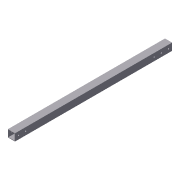
# Autodesk Inventor part: Frame_RearVerticalSupport
Saved by Autodesk Inventor 2012 (Build 160160000, 160)
## iProperties
Created: 2012-01-09
Part Number: Frame_RearVerticalSupport
Material: Aluminum-6061
Document SubType Name: Modeling
Designer: JesseK
Density: 2.71 g/cm^3
Mass: 228.217 g
Surface Area: 1066.35 cm^2
Volume: 84.213 cm^3
Author: JesseK
Autodesk Inventor part; units mm, degrees
ref_plane "YZ Plane" through (0, 0, 0) normal (1, 0, 0) x (0, 1, 0)
ref_plane "XZ Plane" through (0, 0, 0) normal (0, 1, 0) x (-1, 0, 0)
ref_plane "XY Plane" through (0, 0, 0) normal (0, 0, 1) x (1, 0, 0)
sketch "Sketch1" plane through (0, 0, 0) normal (0, 0, 1) x (1, 0, 0)
  line L0 (0, 0) -> (25.4, 0)
  line L1 (25.4, 0) -> (25.4, 25.4)
  line L2 (25.4, 25.4) -> (0, 25.4)
  line L3 (0, 25.4) -> (0, 0)
  dimension "d0" = 25.4
  dimension "d1" = 25.4
  constraints: 8 end point, 2 parallel, 1 horizontal, 1 perpendicular
  measures "d0" distance of L1.end L2.end
  measures "d1" distance of L0.end L1.end
extrude "Extrusion1" add sketch "Sketch1" along normal blind 558.8
shell "Shell1" thickness 1.5875 removed faces 2 at (16.9333, 8.4667, 0) at (16.9333, 8.4667, 558.8)
sketch "Sketch2" plane through (25.4, 0, 0) normal (1, 0, 0) x (0, 0, -1)
  line L0 (-558.8, 25.4) -> (-558.8, 0) projected
  line L1 (0, 25.4) -> (-558.8, 25.4) projected
  circle A0 centre (-546.1, 12.7) radius 2.3813
  circle A1 centre (-520.7, 12.7) radius 2.3813
  dimension "d5" = 12.7
  dimension "d6" = 12.7
  dimension "d7" = 25.4
  dimension "d8" = 12.7
  dimension "d9" = 4.7625
  dimension "d10" = 4.7625
  constraints: 2 centre point
  measures "d5" distance from line of L1 A0.centre
  measures "d6" distance from line of L1 A1.centre
  measures "d7" distance of A1.centre A0.centre
  measures "d8" distance from line of L0 A0.centre
  measures "d9" diameter of A0
  measures "d10" diameter of A1
extrude "Extrusion2" cut sketch "Sketch2" against normal through all
sketch "Sketch3" plane through (25.4, 0, 0) normal (1, 0, 0) x (0, 0, -1)
  line L0 (0, 0) -> (0, 25.4) projected
  line L1 (0, 25.4) -> (-558.8, 25.4) projected
  circle A0 centre (-12.7, 12.7) radius 2.3813
  circle A1 centre (-38.1, 12.7) radius 2.3813
  circle A2 centre (-63.5, 12.7) radius 2.3813
  line L2 (-63.5, 12.7) -> (-38.1, 12.7) construction
  line L3 (-38.1, 12.7) -> (-12.7, 12.7) construction
  dimension "d13" = 12.7
  dimension "d14" = 25.4
  dimension "d15" = 12.7
  dimension "d16" = 4.7625
  constraints: 4 end point, 3 centre point, 2 collinear, 2 equal radius, 1 parallel
  measures "d13" distance from line of L0 L3.end
  measures "d14" distance of L2.end L3.end
  measures "d15" distance between parallel lines of L1 L3
  measures "d16" diameter of A0
extrude "Extrusion3" cut sketch "Sketch3" against normal through all
body "Solid1"
